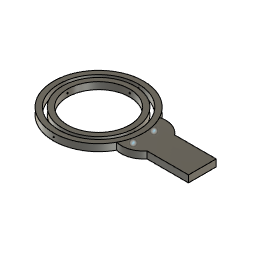
test stand (Autodesk Fusion 360 design; units mm, degrees)
Autodesk Fusion 360 part; units mm, degrees
sketch "Sketch1" plane through (0, 0, 0) normal (0, 0, 1) x (1, 0, 0)
  circle A0 centre (0, 0) radius 45
  circle A1 centre (0, 0) radius 52.5
  dimension "d1" = 90
  dimension "d2" = 105
  constraint coincident A0.centre A1.centre
  constraint concentric A0 A1
  measures "d1" diameter of A0
  measures "d2" diameter of A1
extrude "Extrude1" add sketch "Sketch1" along normal blind 10 makes body 1
sketch "Sketch2" plane through (0, 0, 0) normal (0, 0, 1) x (1, 0, 0)
  circle A0 centre (0, 0) radius 57.5
  circle A1 centre (0, 0) radius 65
  dimension "d5" = 115
  dimension "d6" = 130
  constraint coincident A0.centre A1.centre
  measures "d5" diameter of A0
  measures "d6" diameter of A1
extrude "Extrude2" add sketch "Sketch2" along normal blind 10 separate body makes body 2
sketch "Sketch3" plane through (0, 0, 10) normal (0, 0, 1) x (-1, 0, 0)
  circle A0 centre (0, 0) radius 57.5
  circle A1 centre (0, 0) radius 65
  line L0 (0, 0) -> (0, 65)
  line L1 (0, 0) -> (65, 0)
  line L2 (0, 0) -> (-65, 0)
  constraint coincident A0.centre A1.centre
  constraint coincident A1 L0.end
  constraint vertical L0
  constraint coincident A1 L1.end
  constraint perpendicular L0 L1
  constraint coincident A1 L2.end
  constraint perpendicular L0 L2
ref_plane "WorkPlane1" through (-65, 0, 10) normal (-1, 0, 0) x (0, -1, 0)
sketch "Sketch4" plane through (-65, 0, 0) normal (-1, 0, 0) x (0, -1, 0)
  circle A0 centre (0, 5) radius 1
  dimension "d9" = 2
  measures "d9" diameter of A0
ref_plane "WorkPlane2" through (0, -65, 10) normal (0, -1, 0) x (1, 0, 0)
sketch "Sketch5" plane through (0, -65, 0) normal (0, -1, 0) x (-1, 0, 0)
  circle A0 centre (0, -5) radius 1
  dimension "d10" = 2
  measures "d10" diameter of A0
extrude "Extrude3" cut sketch "Sketch5" against normal blind 195 bodies 1 2
extrude "Extrude4" cut sketch "Sketch4" along normal blind -12 and the other way blind 119 bodies 1
ref_plane "WorkPlane3" through (65, 0, 10) normal (1, 0, 0) x (0, 1, 0)
sketch "Sketch6" plane through (65, 0, 0) normal (1, 0, 0) x (0, 1, 0)
  circle A0 centre (-15, 5) radius 1
  circle A1 centre (15, 5) radius 1
  dimension "d17" = 2
  dimension "d18" = 2
  measures "d17" diameter of A0
  measures "d18" diameter of A1
extrude "Extrude5" cut sketch "Sketch6" along normal up to surface end surface at (8.8883, 56.8089, 4.914) on bodies 2 bodies 2
sketch "Sketch7" plane through (0, 0, 10) normal (0, 0, 1) x (-1, 0, 0)
  circle A0 centre (0, 0) radius 57.5
  circle A1 centre (0, 0) radius 65
  line L0 (-110, 20) -> (-150, 20)
  line L1 (-150, 20) -> (-150, -20)
  line L2 (-150, -20) -> (-90, -20)
  line L3 (-110, 20) -> (-90, 20)
  circle A2 centre (-65, 0) radius 32.0156
  constraint horizontal L0
  constraint perpendicular L0 L1
  constraint perpendicular L1 L2
  constraint parallel L0 L3
  constraint coincident A1 A2.centre
  constraint coincident L2.end A2
extrude "Extrude6" add sketch "Sketch7" against normal up to surface (10 mm away) separate body contours A1 A2 | L0 L1 L2 L3 A2 makes body 3
extrude "Extrude7" cut sketch "Sketch6" along normal blind 15 and the other way blind 5 bodies 3
